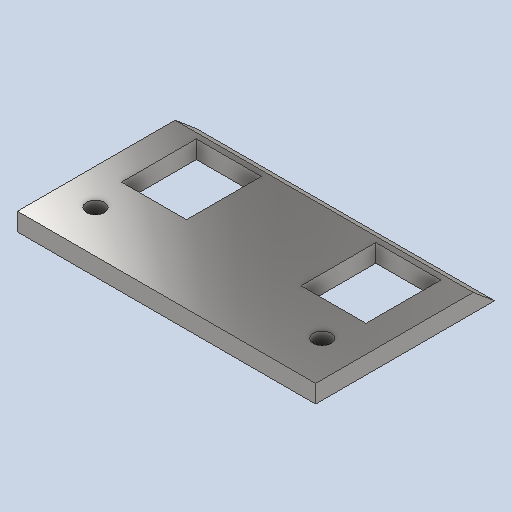
# Autodesk Inventor part: nozz
Saved by Autodesk Inventor 2023 (Build 270158000, 158)
## iProperties
Created: 2023-01-27
Part Number: nozz
Material: Stal nierdzewna
Document SubType Name: Modeling
Designer: Kamil
Density: 8 g/cm^3
Appearance: Częściowo polerowany
Mass: 26.9421 g
Surface Area: 31.3591 cm^2
Volume: 3.36776 cm^3
Author: Kamil
Autodesk Inventor part; units mm, degrees
ref_plane "YZ Plane" through (0, 0, 0) normal (1, 0, 0) x (0, 1, 0)
ref_plane "XZ Plane" through (0, 0, 0) normal (0, 1, 0) x (-1, 0, 0)
ref_plane "XY Plane" through (0, 0, 0) normal (0, 0, 1) x (1, 0, 0)
sketch "Sketch1" plane through (0, 0, 0) normal (1, 0, 0) x (0, 1, 0)
  line L0 (1.944, 4.8709) -> (-1.056, 4.8709)
  line L1 (-1.056, 4.8709) -> (-1.056, -25.1291)
  line L2 (-1.056, -25.1291) -> (1.944, -25.1291)
  line L3 (1.944, -25.1291) -> (1.944, 4.8709)
  line L4 (-1.056, -25.1291) -> (9.6963, -12.315)
  point P0 (0, 0)
  point P1 (1.944, -21.5539)
  dimension "d0" = 3
  dimension "d1" = 30
  dimension "d2" = 40
  constraints: 10 end point, 2 parallel, 1 horizontal, 1 perpendicular
  measures "d0" distance of L2.end L1.end
  measures "d1" distance of L1.end L0.end
  measures "d2" angle of L1 L4
extrude "Extrusion1" add sketch "Sketch1" against normal blind 50 contours L3 L4 L1 L0
sketch "Szkic2" plane through (0, -1.056, -25.1291) normal (0, -1, 0) x (1, 0, 0)
  line L0 (0, 30) -> (0, 0)
  line L1 (0, 30) -> (-50, 30)
  line L2 (-50, 0) -> (-50, 30)
  line L3 (0, 0) -> (-50, 0)
  line L4 (-35.094, 16.557) -> (-35.094, 5.254)
  line L5 (-45, 5) -> (-35.348, 5)
  line L6 (-45, 5) -> (-45, 16.43)
  line L7 (-44.873, 16.557) -> (-35.094, 16.557)
  circle A0 centre (-39.92, 11.35) radius 1
  line L8 (-25, 0) -> (-25, 30)
  line L9 (-35.094, 5.254) -> (-35.348, 5)
  line L10 (-45.5, 16.43) -> (-45.5, 4.5)
  line L11 (-45.5, 4.5) -> (-35.1409, 4.5)
  line L12 (-34.594, 5.0469) -> (-34.594, 17.057)
  line L13 (-34.594, 17.057) -> (-44.873, 17.057)
  line L14 (-35.1409, 4.5) -> (-35.094, 4.5469)
  line L15 (-34.6409, 5) -> (-34.594, 5.0469)
  line L16 (-45.5, 4.5) -> (-34.594, 4.5)
  line L17 (-34.594, 4.5) -> (-34.594, 17.057)
  line L18 (-34.594, 17.057) -> (-45.5, 17.057)
  line L19 (-45.5, 17.057) -> (-45.5, 4.5)
  circle A1 centre (-10.08, 11.35) radius 1
  line L20 (-4.5, 16.43) -> (-4.5, 4.5)
  line L21 (-4.5, 4.5) -> (-14.8591, 4.5)
  line L22 (-15.406, 5.0469) -> (-15.406, 17.057)
  line L23 (-15.406, 17.057) -> (-5.127, 17.057)
  line L24 (-4.5, 4.5) -> (-15.406, 4.5)
  line L25 (-15.406, 4.5) -> (-15.406, 17.057)
  line L26 (-15.406, 17.057) -> (-4.5, 17.057)
  line L27 (-4.5, 17.057) -> (-4.5, 4.5)
  line L28 (0, 4.1492) -> (-50, 4.1492)
  line L29 (-50, 4.1492) -> (-50, 27.66)
  line L30 (-36.5, 27.66) -> (-50, 27.66)
  line L31 (-36.5, 27.66) -> (-36.5, 17.057)
  line L32 (-26.5, 4.66) -> (-36.5, 4.66)
  line L33 (-26.5, 4.66) -> (-26.5, 34.4086)
  line L34 (-23.5, 34.4086) -> (-23.5, 4.66)
  line L35 (-13.5, 4.66) -> (-23.5, 4.66)
  line L36 (-13.5, 4.66) -> (-13.5, 13.5389)
  line L37 (0, 27.66) -> (-13.5, 27.66)
  line L38 (0, 4.1492) -> (0, 27.66)
  line L39 (-50, 4.1492) -> (-44, 4.1492)
  line L40 (-44, 27.66) -> (-50, 27.66)
  line L41 (-50, 27.66) -> (-50, 4.1492)
  line L42 (-50, 27.66) -> (-36.5, 27.66)
  line L43 (-36.5, 27.66) -> (-36.5, 24.66)
  line L44 (-50, 24.66) -> (-50, 27.66)
  circle A2 centre (-10.08, 11.35) radius 1
  circle A3 centre (-39.92, 11.35) radius 1
  line L45 (-6, 27.66) -> (-6, 22.91)
  line L46 (-44, 27.66) -> (-44, 22.91)
  circle A4 centre (-6, 22.91) radius 1.5
  circle A5 centre (-44, 22.91) radius 1.5
  circle A6 centre (-6, 22.91) radius 1.75
  circle A7 centre (-44, 22.91) radius 1.75
  line L47 (-12.975, 17.057) -> (-13.5, 17.057)
  line L48 (-36.5, 17.057) -> (-37.0252, 17.057)
  line L49 (-45.5, 15.557) -> (-45.5, 15.0389)
  line L50 (-37.0252, 13.5389) -> (-36.5, 13.5389)
  line L51 (-36.5, 13.5389) -> (-36.5, 4.66)
  line L52 (-13.5, 13.5389) -> (-12.975, 13.5389)
  line L53 (-4.5, 15.0389) -> (-4.5, 15.557)
  arc A8 (-12, 17.057) -> (-12.975, 16.6969) centre (-12, 15.557) ccw
  line L54 (-12.975, 16.6969) -> (-12.975, 17.057)
  line L55 (-37.0252, 16.697) -> (-37.0252, 17.057)
  arc A9 (-37.0252, 16.697) -> (-38, 17.057) centre (-38, 15.557) ccw
  arc A10 (-44, 17.057) -> (-45.5, 15.557) centre (-44, 15.557) ccw
  arc A11 (-45.5, 15.0389) -> (-44, 13.5389) centre (-44, 15.0389) ccw
  arc A12 (-38, 13.5389) -> (-37.0252, 13.8988) centre (-38, 15.0389) ccw
  line L56 (-37.0252, 13.8988) -> (-37.0252, 13.5389)
  line L57 (-12.975, 13.899) -> (-12.975, 13.5389)
  arc A13 (-12.975, 13.899) -> (-12, 13.5389) centre (-12, 15.0389) ccw
  line L58 (-12, 13.5389) -> (-6, 13.5389)
  arc A14 (-6, 13.5389) -> (-4.5, 15.0389) centre (-6, 15.0389) ccw
  arc A15 (-4.5, 15.557) -> (-6, 17.057) centre (-6, 15.557) ccw
  line L59 (-6, 17.057) -> (-12, 17.057)
  line L60 (-38, 17.057) -> (-44, 17.057)
  line L61 (-44, 13.5389) -> (-38, 13.5389)
  arc A16 (-26.5, 34.4086) -> (-23.5, 34.4086) centre (-25, 35.31) ccw
  line L62 (-13.5, 17.057) -> (-13.5, 27.66)
  point P0 (0, 25.1291)
  point P1 (-45.5, 13.5389)
  point P2 (-4.5, 13.5389)
extrude "Wyciągnięcie proste2" cut sketch "Szkic2" against normal through all contours L35 L36 L52 L57 A13 L58 A14 L20 L21 L24 L25 | L25 L22 L23 L54 A8 A15 L20 A14 L58 A13 L57 L52 L36 L35 | L23 A8 L54 | L32 L51 L50 L56 A12 L61 A11 L10 A10 L13 A9 L55 L12 L17 | L17 L16 L11 L10 A11 L6 L5 L51 L32 | L23 L26 L27 L20 A15 | L5 L6 A11 L61 A12 L56 L50 L51 | L55 A9 L13 | L10 L19 L18 L13 A10 | A0 | A1
sketch "Szkic3" plane through (0, -1.056, -25.1291) normal (0, -1, 0) x (1, 0, 0)
  line L0 (-4.5, 17.057) -> (-4.5, 4.5) projected
  line L1 (-4.5, 4.5) -> (-15.406, 4.5) projected
  line L2 (-15.406, 4.5) -> (-15.406, 17.057) projected
  line L3 (-15.406, 17.057) -> (-4.5, 17.057) projected
  line L4 (-34.594, 17.057) -> (-34.594, 4.5) projected
  line L5 (-34.594, 4.5) -> (-45.5, 4.5) projected
  line L6 (-45.5, 4.5) -> (-45.5, 17.057) projected
  line L7 (-45.5, 17.057) -> (-34.594, 17.057) projected
  line L8 (0, 30) -> (0, 0) projected
  line L9 (0, 30) -> (-50, 30) projected
  line L10 (-50, 0) -> (-50, 30) projected
  line L11 (0, 0) -> (-50, 0) projected
  circle A0 centre (-44, 24.66) radius 1.75 projected
  circle A1 centre (-10.08, 11.35) radius 1 projected
  circle A2 centre (-39.92, 11.35) radius 1 projected
  line L12 (0, 4.1492) -> (-50, 4.1492) projected
  line L13 (-50, 4.1492) -> (-50, 27.66) projected
  line L14 (-36.5, 27.66) -> (-50, 27.66) projected
  line L15 (-36.5, 27.66) -> (-36.5, 17.057) projected
  line L16 (-26.5, 4.66) -> (-36.5, 4.66) projected
  line L17 (-26.5, 4.66) -> (-26.5, 34.4086) projected
  line L18 (-23.5, 34.4086) -> (-23.5, 4.66) projected
  line L19 (-13.5, 4.66) -> (-23.5, 4.66) projected
  line L20 (-13.5, 4.66) -> (-13.5, 13.5389) projected
  line L21 (0, 27.66) -> (-13.5, 27.66) projected
  line L22 (0, 4.1492) -> (0, 27.66) projected
  line L23 (-44, 27.66) -> (-44, 22.91)
  line L24 (-6, 27.66) -> (-6, 22.91)
  circle A3 centre (-44, 22.91) radius 1.5
  circle A4 centre (-6, 22.91) radius 1.5
  circle A5 centre (-6, 22.91) radius 1.75 projected
  circle A6 centre (-44, 22.91) radius 1.75 projected
  line L25 (-12.975, 17.057) -> (-13.5, 17.057) projected
  line L26 (-36.5, 17.057) -> (-37.0252, 17.057) projected
  line L27 (-45.5, 15.557) -> (-45.5, 15.0389) projected
  line L28 (-37.0252, 13.5389) -> (-36.5, 13.5389) projected
  line L29 (-36.5, 13.5389) -> (-36.5, 4.66) projected
  line L30 (-13.5, 13.5389) -> (-12.975, 13.5389) projected
  line L31 (-4.5, 15.0389) -> (-4.5, 15.557) projected
  arc A7 (-12, 17.057) -> (-12.975, 16.6969) centre (-12, 15.557) ccw projected
  line L32 (-12.975, 16.6969) -> (-12.975, 17.057) projected
  line L33 (-37.0252, 16.697) -> (-37.0252, 17.057) projected
  arc A8 (-37.0252, 16.697) -> (-38, 17.057) centre (-38, 15.557) ccw projected
  arc A9 (-44, 17.057) -> (-45.5, 15.557) centre (-44, 15.557) ccw projected
  arc A10 (-45.5, 15.0389) -> (-44, 13.5389) centre (-44, 15.0389) ccw projected
  arc A11 (-38, 13.5389) -> (-37.0252, 13.8988) centre (-38, 15.0389) ccw projected
  line L34 (-37.0252, 13.8988) -> (-37.0252, 13.5389) projected
  line L35 (-12.975, 13.899) -> (-12.975, 13.5389) projected
  arc A12 (-12.975, 13.899) -> (-12, 13.5389) centre (-12, 15.0389) ccw projected
  line L36 (-12, 13.5389) -> (-6, 13.5389) projected
  arc A13 (-6, 13.5389) -> (-4.5, 15.0389) centre (-6, 15.0389) ccw projected
  arc A14 (-4.5, 15.557) -> (-6, 17.057) centre (-6, 15.557) ccw projected
  line L37 (-6, 17.057) -> (-12, 17.057) projected
  line L38 (-38, 17.057) -> (-44, 17.057) projected
  line L39 (-44, 13.5389) -> (-38, 13.5389) projected
  arc A15 (-26.5, 34.4086) -> (-23.5, 34.4086) centre (-25, 35.31) ccw projected
  line L40 (-13.5, 17.057) -> (-13.5, 27.66) projected
  point P0 (0, 25.1291)
  point P1 (-45.5, 13.5389)
  point P2 (-4.5, 13.5389)
  dimension "d13" = 3
  dimension "d14" = 3
  constraints: 4 end point, 2 centre point, 2 coincident, 2 point on line, 1 perpendicular
  measures "d13" diameter of A3
  measures "d14" diameter of A4
extrude "Wyciągnięcie proste3" cut sketch "Szkic3" against normal through all contours A4 | A3 L23 A0 | A0 A3 | A3 A0 L23
body "Solid1"
